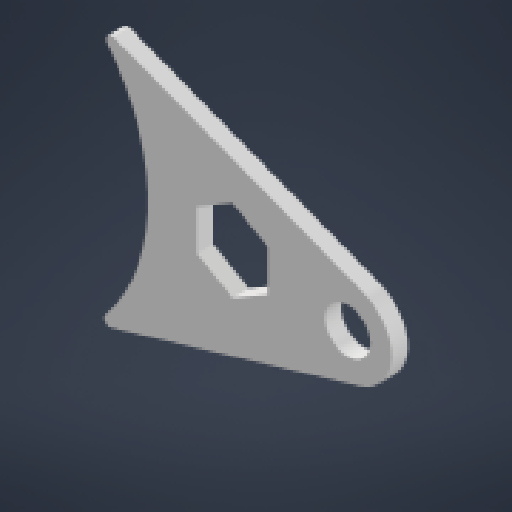
# Autodesk Inventor part: gear-interface
Saved by Autodesk Inventor 2023.2 (Build 272271000, 271)
## iProperties
Created: 2023-03-20
Part Number: gear-interface
Material: Generic
Document SubType Name: Modeling
Designer: Liam
Density: 1 g/cm^3
Appearance: Default
Author: Liam
Autodesk Inventor part; units mm, degrees
ref_plane "YZ Plane" through (0, 0, 0) normal (1, 0, 0) x (0, 1, 0)
ref_plane "XZ Plane" through (0, 0, 0) normal (0, 1, 0) x (-1, 0, 0)
ref_plane "XY Plane" through (0, 0, 0) normal (0, 0, 1) x (1, 0, 0)
sketch "Sketch1" plane through (0, 0, 0) normal (0, 0, 1) x (1, 0, 0)
  circle A0 centre (12.6998, -0.0001) radius 2.0955 projected
  circle A1 centre (12.6998, -0.0001) radius 3.6662
  line L0 (25.3998, 3.8099) -> (28.6994, 1.9049)
  line L1 (28.6994, -1.9051) -> (28.6994, 1.9049)
  line L2 (28.6994, -1.9051) -> (25.3998, -3.8101)
  line L3 (22.1003, -1.9051) -> (25.3998, -3.8101)
  line L4 (22.1003, -1.9051) -> (22.1003, 1.9049)
  line L5 (25.3998, 3.8099) -> (22.1003, 1.9049)
  circle A2 centre (36.114, -1.1018) radius 2.0955 projected
  arc A3 (13.5875, -11.0697) -> (17.526, -0.0001) centre (0, 0) ccw
  arc A4 (12.3927, -12.3928) -> (13.7615, 10.8527) centre (0, 0) ccw
  line L6 (37.5751, 2.6904) -> (14.3431, 11.6413)
  line L7 (37.272, -4.9974) -> (14.1261, -11.8776)
  arc A5 (14.3431, 11.6413) -> (13.7615, 10.8527) centre (14.1604, 11.1673) ccw
  arc A6 (13.5875, -11.0697) -> (14.1261, -11.8776) centre (13.9814, -11.3906) ccw
  arc A7 (37.272, -4.9974) -> (37.5751, 2.6904) centre (36.114, -1.1018) ccw
  point P0 (12.6998, 3.6661)
  point P1 (16.4691, 5.9941)
  point P2 (16.469, -5.9943)
  point P3 (30.4798, 5.0799)
  point P4 (30.4798, -5.0801)
  point P5 (12.3928, 12.3927)
  point P6 (12.3927, -12.3928)
  point P7 (17.526, -0.0001)
  dimension "d28" = 0.508
  constraints: 16 end point, 12 point on circle, 5 centre point, 4 tangent, 3 parallel, 3 vertical, 2 coincident, 2 point on line, 1 equal radius, 1 vertical alignment, 8 other
  measures "d28" radius of A5
extrude "Extrusion3" add sketch "Sketch1" along normal blind 1.524 contours A3 A4 A5 L6 A7 L7 A6
body "Solid3"
